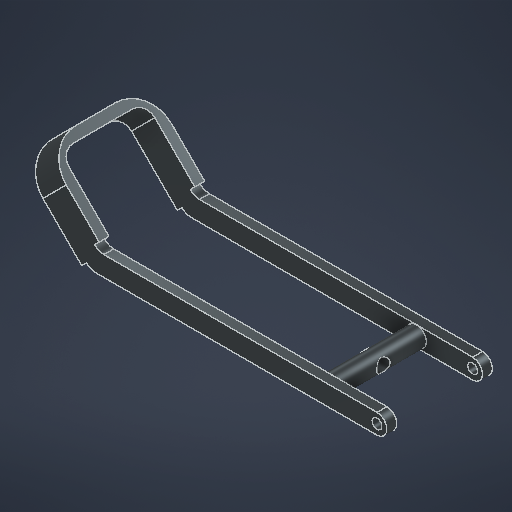
# Autodesk Inventor part: BODY-220LB
Saved by Autodesk Inventor 2025.3 (Build 293356030, 356C)
## iProperties
Created: 2025-08-31
Part Number: BODY-220LB
Material: Generic
Document SubType Name: Modeling
Designer: lstk1ng
Density: 1 g/cm^3
Appearance: Iron Gray
Author: lstk1ng
Autodesk Inventor part; units mm, degrees
ref_plane "YZ Plane" through (0, 0, 0) normal (1, 0, 0) x (0, 1, 0)
ref_plane "XZ Plane" through (0, 0, 0) normal (0, 1, 0) x (-1, 0, 0)
ref_plane "XY Plane" through (0, 0, 0) normal (0, 0, 1) x (1, 0, 0)
sketch "Sketch1" plane through (0, 0, 0) normal (0, 0, 1) x (1, 0, 0)
  line L0 (0, 0) -> (55, 0)
  line L1 (55, 0) -> (10, 0)
  line L2 (10, 0) -> (0, 10)
  line L3 (0, 10) -> (2.1213, 12.1213)
  line L4 (2.1213, 12.1213) -> (10, 4.2426)
  line L5 (55, 0) -> (55, 3)
  line L6 (55, 3) -> (11.2426, 3)
  line L7 (11.2426, 3) -> (10, 4.2426)
  dimension "d0" = 55
  dimension "d1" = 45
  dimension "d2" = 135
  dimension "d3" = 3
  dimension "d4" = 3
  constraints: 16 end point, 3 perpendicular, 2 point on line, 1 horizontal, 1 vertical
  measures "d0" distance of L0.start L0.end
  measures "d1" distance of L0.end L1.end
  measures "d2" angle of L1 L2
  measures "d3" distance of L2.end L3.end
  measures "d4" distance of L0.end L5.end
extrude "Extrusion1" add sketch "Sketch1" along normal blind 16
sketch "Sketch2" plane through (2.1213, 12.1213, 0) normal (0.7071068, 0.7071068, 0) x (-0.7071068, 0.7071068, 0)
  line L0 (-12.8995, 0) -> (-12.8995, 16) projected
  line L1 (-1.5, 12.5) -> (-1.5, 3.5)
  line L2 (-3.5, 1.5) -> (-11.3995, 1.5)
  line L3 (-11.3995, 14.5) -> (-3.5, 14.5)
  line L4 (-11.3995, 14.5) -> (-12.8995, 14.5)
  line L5 (-11.3995, 1.5) -> (-12.8995, 1.5)
  arc A0 (-1.5, 12.5) -> (-3.5, 14.5) centre (-3.5, 12.5) ccw
  arc A1 (-3.5, 1.5) -> (-1.5, 3.5) centre (-3.5, 3.5) ccw
  point P0 (-7.0711, 0)
  dimension "d7" = 2
  constraints: 10 end point, 4 point on circle, 4 tangent, 2 centre point, 2 perpendicular, 2 point on line, 1 equal radius
  measures "d7" radius of A0
extrude "Extrusion2" cut sketch "Sketch2" against normal up to surface (3 mm away)
sketch "Sketch3" plane through (11.2426, 3, 0) normal (0, 1, 0) x (1, 0, 0)
  line L0 (42.7574, -15) -> (43.7574, -15)
  line L1 (43.7574, -15) -> (43.7574, -1.5)
  line L2 (43.7574, 0) -> (43.7574, -16) projected
  line L3 (-2.1213, -14.5) -> (-2.1213, -1.5) projected
  line L4 (-2.1213, -14.5) -> (-2.1213, -1.5)
  line L5 (0, -1.5) -> (-2.1213, -1.5) projected
  line L6 (-2.1213, -1.5) -> (43.7574, -1.5)
  line L7 (-2.1213, -14.5) -> (43.7574, -14.5)
  point P0 (43.7574, -1)
  constraints: 10 end point, 4 point on line, 2 perpendicular, 1 collinear, 1 horizontal
extrude "Extrusion3" cut sketch "Sketch3" against normal up to surface (3 mm away)
fillet "Fillet1" radius 1.5 4 edges at (55, 3, 0.75) (55, 3, 15.25) (55, 0, 0.75) (55, 0, 15.25)
sketch "Sketch5" plane through (53.5, 0, 14.5) normal (0, 0, -1) x (-1, 0, 0)
  arc A0 (0, 3) -> (0, 0) centre (0, 1.5) ccw projected
  line L0 (-1.5, 1.5) -> (8.5, 1.5) construction
  circle A1 centre (8.5, 1.5) radius 1.5
  line L1 (0, 3) -> (42.2574, 3) projected
  point P0 (53.5, 0)
  dimension "d16" = 10
  constraints: 2 end point, 1 centre point, 1 coincident, 1 horizontal, 1 point on circle, 1 tangent
  measures "d16" distance of L0.start L0.end
extrude "Extrusion5" add sketch "Sketch5" along normal up to surface (13 mm away)
fillet "Fillet2" radius 2 4 edges at (10, 0, 15.25) (11.2426, 3, 15.25) (11.2426, 3, 0.75) (10, 0, 0.75)
fillet "Fillet3" radius 5 2 edges at (1.0607, 11.0607, 16) (1.0607, 11.0607, 0)
thicken "Thicken1" operation add thickness 1 both sides no extend neighbours no toward (-0.7071068, -0.7071068, 0) faces at (5.1415, 4.8585, 15)
thicken "Thicken2" operation add thickness 1 both sides no extend neighbours no toward (0.7071068, 0.7071068, 0) faces at (2.8284, 11.4142, 7)
sketch "Sketch6" plane through (0, 0, 16) normal (0, 0, 1) x (1, 0, 0)
  arc A0 (53.5, 0) -> (53.5, 3) centre (53.5, 1.5) ccw projected
  circle A1 centre (53.5, 1.5) radius 0.75
  point P0 (0, 0)
  dimension "d25" = 1.5
  constraints: 1 centre point, 1 coincident
  measures "d25" diameter of A1
extrude "Extrusion6" cut sketch "Sketch6" against normal up to surface (16 mm away)
sketch "Sketch7" plane through (0, 0, 0) normal (1, 0, 0) x (0, 1, 0)
  line L0 (5.7574, 0) -> (-0.1213, 0) projected
  line L1 (5.7574, 16) -> (-0.1213, 16) projected
  circle A0 centre (1.5, 8) radius 1
  point P0 (0, 0)
  point P1 (3, 1.5)
  dimension "d28" = 2
  dimension "d29" = 8
  dimension "d30" = 1.5
  constraints: 1 centre point
  measures "d28" diameter of A0
  measures "d29" distance from line of L1 A0.centre
  measures "d30" horizontal distance of point (3, 1.5) A0.centre
extrude "Extrusion7" cut sketch "Sketch7" along normal through all
body "Solid1"
